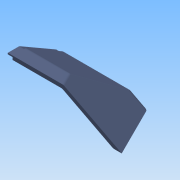
# Autodesk Inventor part: термокрышка
Saved by Autodesk Inventor 2017 (Build 210142000, 142)
## iProperties
Part Number: термокрышка
Material: Типовые
Document SubType Name: Modeling
Designer: Max
Density: 1 g/cm^3
Appearance: Резина — синяя
Mass: 50.9023 g
Surface Area: 230.86 cm^2
Volume: 50.9023 cm^3
Author: Max
Autodesk Inventor part; units mm, degrees
ref_plane "YZ Plane" through (0, 0, 0) normal (1, 0, 0) x (0, 1, 0)
ref_plane "XZ Plane" through (0, 0, 0) normal (0, 1, 0) x (-1, 0, 0)
ref_plane "XY Plane" through (0, 0, 0) normal (0, 0, 1) x (1, 0, 0)
sketch "Эскиз2" plane through (0, 0, 0) normal (0, 0, 1) x (1, 0, 0)
  circle A0 centre (181, -158) radius 2 projected
  circle A1 centre (-181, 158) radius 2 projected
  circle A2 centre (181, 158) radius 2 projected
  circle A3 centre (-181, -158) radius 2 projected
  circle A4 centre (15.5, 126.5) radius 1.5 projected
  circle A5 centre (-15.5, 157.5) radius 1.5 projected
  circle A6 centre (15.5, 157.5) radius 1.5 projected
  circle A7 centre (-15.5, 126.5) radius 1.5 projected
  line L0 (89, 108) -> (89, 96) projected
  line L1 (89, 96) -> (69, 96) projected
  line L2 (69, 96) -> (69, 108) projected
  line L3 (69, 108) -> (89, 108) projected
  line L4 (168.6, 126.6) -> (168.6, 100.6) projected
  line L5 (168.6, 100.6) -> (140.6, 100.6) projected
  line L6 (140.6, 100.6) -> (140.6, 126.6) projected
  line L7 (140.6, 126.6) -> (168.6, 126.6) projected
  circle A8 centre (-92.5, 142) radius 6 projected
  circle A9 centre (-103.5, 142) radius 1.5 projected
  circle A10 centre (103.5, 142) radius 1.5 projected
  circle A11 centre (81.5, 142) radius 1.5 projected
  circle A12 centre (-81.5, 142) radius 1.5 projected
  circle A13 centre (92.5, 142) radius 6 projected
  circle A14 centre (0, 142) radius 11.5 projected
  line L8 (-107.3915, -104.3944) -> (-139.1034, -168)
  line L9 (107.3915, -104.3944) -> (-107.3915, -104.3944) projected
  line L10 (139.1034, -168) -> (107.3915, -104.3944)
  line L11 (189, 166) -> (189, -166) projected
  line L12 (-189, 166) -> (189, 166) projected
  line L13 (-189, -166) -> (-189, 166) projected
  line L14 (189, -168) -> (-189, -168) projected
  line L15 (-184, -161) -> (-184, 161)
  line L16 (-184, 161) -> (184, 161)
  line L17 (184, 161) -> (184, -161)
  line L18 (144.6904, -168) -> (110.4856, -99.3944)
  line L19 (110.4856, -99.3944) -> (-110.4856, -99.3944)
  line L20 (-110.4856, -99.3944) -> (-144.6904, -168)
  line L21 (-144.6904, -168) -> (144.6904, -168)
  point P0 (0, 0)
  dimension "d9" = 5
  constraints: 18 end point, 4 point on line, 1 collinear, 2 other
  measures "d9" distance between parallel lines of L8 L20
extrude "Выдавливание1" add sketch "Эскиз2" along normal blind 50 contours L9 L10 L14 L8 | L8 L14 L20 L19 L18 L10 L9
sketch "Эскиз4" plane through (-144.6904, -168, 0) normal (0, -1, 0) x (1, 0, 0)
  line L0 (59.1192, 66.315) -> (219.6093, 66.315)
  line L1 (219.6093, 66.315) -> (219.6093, 40)
  line L2 (219.6093, 40) -> (59.1192, 40)
  line L3 (59.1192, 40) -> (59.1192, 66.315)
  line L4 (0, 0) -> (289.3807, 0) projected
  point P0 (144.6904, 0)
  dimension "d20" = 40
  constraints: 8 end point, 2 parallel, 1 horizontal, 1 perpendicular
  measures "d20" distance between parallel lines of L4 L2
draft "НаклГрань6" angle 30 pull direction (0, 1, 0) faces at (36.8285, -145.1315, 50) fixed edges at (0, -168, 50)
draft "НаклГрань7" angle 60 pull direction (0, 0, 1) faces at (133.2888, -145.1315, 20.1302) fixed edges at (127.588, -133.6972, 0)
draft "НаклГрань8" angle 60 pull direction (0, 0, 1) faces at (-133.2888, -145.1315, 20.1302) fixed edges at (-127.588, -133.6972, 0)
extrude "Выдавливание3" cut sketch "Эскиз4" against normal blind 60
shell "Оболочка1" thickness 5 removed faces 2 at (-22.425, -168, 13.3333) at (36.8285, -145.1315, 0)
fillet "Сопряжение1" radius 5 2 edges at (-117.6605, -136.1972, 0) (117.6605, -136.1972, 0)
fillet "Сопряжение2" radius 5 9 edges at (-72.5461, -128.2068, 21.2519) (-101.8555, -104.3944, 0.1704) (-93.8949, -104.3944, 4.0868) (0, -104.3944, 7.5038) (0, -152.0192, 35) (-61.7941, -160.0096, 35) (61.7941, -160.0096, 35) (72.5461, -128.2068, 21.2519) (93.8949, -104.3944, 4.0868)
fillet "Сопряжение3" radius 5 8 edges at (62.9572, -159.3397, 40) (-62.9572, -159.3397, 40) (0, -150.6795, 40) (-74.5077, -125.037, 25.1953) (74.5077, -125.037, 25.1953) (100.4308, -99.3944, 5.1953) (0, -99.3944, 10.3906) (-100.4308, -99.3944, 5.1953)
sketch "Эскиз6" plane through (-144.6904, -168, 0) normal (0, -1, 0) x (1, 0, 0)
  line L0 (144.6904, 0) -> (-83.4893, 0)
  line L1 (-83.4893, 0) -> (-83.4893, 70.7931)
  line L2 (-83.4893, 70.7931) -> (144.6904, 70.7931)
  line L3 (144.6904, 70.7931) -> (144.6904, 0)
  line L4 (32.268, 0) -> (0, 0) projected
  dimension "d38" = 144.6904
  constraints: 8 end point, 2 parallel, 1 horizontal, 1 perpendicular
  measures "d38" distance from line of L3 L4.end
extrude "Выдавливание4" cut sketch "Эскиз6" against normal blind 200
sketch "Эскиз7" plane through (0, -168, 35) normal (-1, 0, 0) x (0, 0, 1)
  line L0 (-35, 68.6056) -> (-27.4962, 68.6056) projected
  line L1 (-35, 63.6056) -> (-35, 68.6056) projected
  line L2 (-30.3829, 63.6056) -> (-35, 63.6056) projected
  arc A0 (-26.0528, 61.1056) -> (-30.3829, 63.6056) centre (-30.3829, 58.6056) ccw projected
  line L3 (-0.6699, 17.141) -> (-26.0528, 61.1056) projected
  arc A1 (0, 14.641) -> (-0.6699, 17.141) centre (-5, 14.641) ccw projected
  line L4 (0, 0) -> (0, 14.641) projected
  line L5 (5, 0) -> (0, 0) projected
  line L6 (5, 15.9808) -> (5, 0) projected
  arc A2 (5, 15.9808) -> (4.3301, 18.4808) centre (0, 15.9808) ccw projected
  line L7 (-23.1661, 66.1056) -> (4.3301, 18.4808) projected
  arc A3 (-23.1661, 66.1056) -> (-27.4962, 68.6056) centre (-27.4962, 63.6056) ccw projected
  arc A4 (3.35, 15.9808) -> (2.9012, 17.6558) centre (0, 15.9808) ccw
  line L8 (3.35, 15.9808) -> (3.35, 1.65)
  line L9 (3.35, 1.65) -> (1.65, 1.65)
  line L10 (1.65, 1.65) -> (1.65, 14.641)
  arc A5 (1.65, 14.641) -> (0.7591, 17.966) centre (-5, 14.641) ccw
  line L11 (0.7591, 17.966) -> (-24.6239, 61.9306)
  arc A6 (-24.6239, 61.9306) -> (-30.3829, 65.2556) centre (-30.3829, 58.6056) ccw
  line L12 (-30.3829, 65.2556) -> (-33.35, 65.2556)
  line L13 (-33.35, 65.2556) -> (-33.35, 66.9556)
  line L14 (-33.35, 66.9556) -> (-27.4962, 66.9556)
  arc A7 (-24.595, 65.2806) -> (-27.4962, 66.9556) centre (-27.4962, 63.6056) ccw
  line L15 (-24.595, 65.2806) -> (2.9012, 17.6558)
  point P0 (-35, 168)
  dimension "d41" = 1.65
  constraints: 16 end point, 8 point on circle, 4 centre point, 11 other
  measures "d41" distance between parallel lines of L7 L15
extrude "Выдавливание5" add sketch "Эскиз7" along normal blind 4 contours L8 L9 L10 A5 L11 A6 L12 L13 L14 A7 L15 A4
